Back Extention (Autodesk Fusion 360 design; units mm, degrees)
Autodesk Fusion 360 part; units mm, degrees
sketch "Sketch1" plane through (0, 0, 0) normal (0, 0, 1) x (1, 0, 0)
  line L0 (0, 0) -> (0, 121.8)
  line L1 (0, 0) -> (78.294095, 20.97884)
  line L2 (82, 25.808469) -> (82, 176.135475)
  line L3 (82, 176.135475) -> (44, 176.135475)
  line L4 (44, 176.135475) -> (0, 121.8)
  arc A0 (78.294095, 20.97884) -> (82, 25.808469) centre (77, 25.808469) ccw
  line L5 (3, 3.909676) -> (77.517638, 23.876617)
  arc A1 (77.517638, 23.876617) -> (79, 25.808469) centre (77, 25.808469) ccw
  line L6 (79, 25.808469) -> (79, 173.135475)
  line L7 (79, 173.135475) -> (45.430927, 173.135475)
  line L8 (45.430927, 173.135475) -> (3, 120.737644)
  line L9 (3, 3.909676) -> (3, 120.737644)
  line L10 (3, 91.254041) -> (79, 91.254041) construction
  line L11 (41, 167.663736) -> (41, 14.091745) construction
  circle A2 centre (41, 128.135475) radius 5
  circle A3 centre (41, 45) radius 5
  dimension "d3" = 121.8
  dimension "d4" = 75
  dimension "d5" = 141
  dimension "d6" = 82
  dimension "d7" = 75
  dimension "d8" = 38
  dimension "d9" = 5
  dimension "d64" = -3
  dimension "d86" = 10
  dimension "d87" = 45
  dimension "d88" = 10
  dimension "d89" = 45
  constraint coincident L0.start L1.start
  constraint vertical L0
  constraint parallel L0 L2
  constraint perpendicular L0 L3
  constraint tangent L2 A0
  constraint tangent L1 A0
  constraint perpendicular L6 L10
  constraint perpendicular L10 L11
  constraint coincident L11 A3.centre
  measures "d3" distance of L0.start L0.end
  measures "d4" angle of L0 L1
  measures "d5" angle of L0 L4
  measures "d6" distance of L0 L2
  measures "d7" angle of L0 L1
  measures "d9" radius of A0
  measures "d86" diameter of A2
  measures "d88" diameter of A3
  measures "d89" vertical distance of L0.start A3.centre
extrude "Extrude7" add sketch "Sketch1" along normal blind 3 contours L5 A1 L6 L7 L8 L9 | A2 | A3 picked at (67.925955, 108.535214) picked at (43.631771, 126.680026) picked at (42.542117, 43.337994) makes body 1
extrude "Extrude13" add sketch "Sketch1" along normal blind 45 contours L0 L1 L2 L3 L4 A0 | A2 | A3 picked at (81, 125.026473) picked at (43.631771, 126.680026) picked at (42.542117, 43.337994) bodies 1
sketch "Sketch2" plane through (0, 0, 0) normal (-1, 0, 0) x (0, -1, 0)
  line L0 (-121.8, 0) -> (0, 0)
  line L1 (0, 0) -> (0, 45)
  line L2 (0, 45) -> (-121.8, 45)
  line L3 (-121.8, 45) -> (-121.8, 0)
  line L4 (-45.9, 42) -> (-75.9, 42)
  line L5 (-75.9, 42) -> (-75.9, 6)
  line L6 (-75.9, 6) -> (-45.9, 6)
  line L7 (-45.9, 6) -> (-45.9, 42)
  line L8 (-45.9, 42) -> (-75.9, 6) construction
  line L9 (-75.9, 42) -> (-45.9, 6) construction
  line L10 (-60.9, 45) -> (-60.9, 0) construction
  line L11 (-30.9, 39) -> (-90.9, 39) construction
  line L12 (-90.9, 39) -> (-90.9, 9) construction
  line L13 (-90.9, 9) -> (-30.9, 9) construction
  line L14 (-30.9, 9) -> (-30.9, 39) construction
  line L15 (-30.9, 39) -> (-90.9, 9) construction
  line L16 (-90.9, 39) -> (-30.9, 9) construction
  circle A0 centre (-90.9, 9) radius 2.1
  circle A1 centre (-90.9, 39) radius 2.1
  circle A2 centre (-30.9, 9) radius 2.1
  circle A3 centre (-30.9, 39) radius 2.1
  line L17 (0, 29.417) -> (-121.8, 29.417) construction
  circle A4 centre (-10, 29.417) radius 5
  circle A5 centre (-111.8, 29.417) radius 5
  line L18 (-121.8, 0) -> (0, 0)
  line L19 (0, 0) -> (0, 45)
  line L20 (0, 45) -> (-121.8, 45)
  line L21 (-121.8, 45) -> (-121.8, 0)
  point P0 (-60.9, 24)
  point P1 (-60.9, 24)
  dimension "d16" = 30
  dimension "d17" = 36
  dimension "d19" = 60
  dimension "d20" = 30
  dimension "d21" = 4.2
  dimension "d22" = 4.2
  dimension "d23" = 4.2
  dimension "d24" = 4.2
  dimension "d26" = 50.9
  dimension "d27" = 10
  dimension "d54" = 30.9
  dimension "d55" = 90.9
  dimension "d67" = 29.417
  dimension "d68" = 6
  constraint horizontal L4
  constraint perpendicular L4 L5
  constraint parallel L4 L6
  constraint parallel L5 L7
  constraint coincident L8 P1
  constraint coincident L9 P1
  constraint midpoint L2 L10.start
  constraint midpoint L0 L10.end
  constraint coincident P1 L10
  constraint horizontal L11
  constraint perpendicular L11 L12
  constraint parallel L11 L13
  constraint parallel L12 L14
  constraint coincident L15 P1
  constraint coincident L16 P1
  constraint coincident P1 P0
  constraint coincident L12.end L13.start
  constraint coincident L11.end L12.start
  constraint coincident L13.end L14.start
  constraint coincident L11.start L14.end
  constraint coincident L1 L17.start
  constraint coincident L3 L17.end
  constraint perpendicular L3 L17
  constraint coincident L17 A4.centre
  constraint symmetric L10 A4 A5
  measures "d16" distance of L5.end L6.end
  measures "d17" distance of L4.end L5.end
  measures "d19" distance of L12.end L13.end
  measures "d20" distance of L11.end L12.end
  measures "d21" diameter of A0
  measures "d22" diameter of A1
  measures "d23" diameter of A2
  measures "d24" diameter of A3
  measures "d26" distance of L10 A4.centre
  measures "d27" diameter of A4
  measures "d54" horizontal distance of L0.end L13.end
  measures "d55" horizontal distance of L0.end L12.end
  measures "d67" distance of L0.end L17.start
  measures "d68" vertical distance of L0.end L6.end
extrude "Extrude16" cut sketch "Sketch2" against normal blind 10 contours L4 L5 L6 L7 | A0 | A1 | A2 | A3 | A4 | A5 picked at (-65.9, 18) picked at (-90.207818, 8.89567) picked at (-91.354622, 39.606218) picked at (-32.17464, 9.251722) picked at (-31.534769, 38.918203) picked at (-10.833333, 30.579729) picked at (-113.210608, 28.925741) bodies 1
sketch "Sketch3" plane through (0, 176.135475, 0) normal (0, 1, 0) x (-1, 0, 0)
  line L0 (-82, 0) -> (-44, 0)
  line L1 (-44, 0) -> (-44, 45)
  line L2 (-44, 45) -> (-82, 45)
  line L3 (-82, 45) -> (-82, 0)
  line L4 (-44, 45) -> (-82, 0) construction
  line L5 (-50.5, 7.5) -> (-75.5, 7.5) construction
  line L6 (-75.5, 7.5) -> (-75.5, 37.5) construction
  line L7 (-75.5, 37.5) -> (-50.5, 37.5) construction
  line L8 (-50.5, 37.5) -> (-50.5, 7.5) construction
  line L9 (-50.5, 7.5) -> (-75.5, 37.5) construction
  line L10 (-75.5, 7.5) -> (-50.5, 37.5) construction
  circle A0 centre (-75.5, 37.5) radius 1.6
  circle A1 centre (-50.5, 37.5) radius 1.6
  circle A2 centre (-75.5, 7.5) radius 1.6
  circle A3 centre (-50.5, 7.5) radius 1.6
  circle A4 centre (-63, 22.5) radius 12.5
  line L11 (-82, 0) -> (-44, 0)
  line L12 (-44, 0) -> (-44, 45)
  line L13 (-44, 45) -> (-82, 45)
  line L14 (-82, 45) -> (-82, 0)
  point P0 (-63, 22.5)
  dimension "d30" = 3.2
  dimension "d31" = 3.2
  dimension "d32" = 3.2
  dimension "d33" = 3.2
  dimension "d34" = 25
  dimension "d35" = 30
  dimension "d36" = 25
  constraint coincident L1.end L2.start
  constraint coincident L0.start L3.end
  constraint horizontal L5
  constraint perpendicular L5 L6
  constraint parallel L5 L7
  constraint parallel L6 L8
  constraint coincident L9 P0
  constraint coincident L10 P0
  constraint midpoint L4 P0
  constraint coincident L6.end L7.start
  constraint coincident L7.end L8.start
  constraint coincident L5.end L6.start
  constraint coincident L5.start L8.end
  constraint coincident P0 A4.centre
  measures "d30" diameter of A0
  measures "d31" diameter of A1
  measures "d32" diameter of A2
  measures "d33" diameter of A3
  measures "d34" distance of L6.end L7.end
  measures "d35" distance of L5.end L6.end
  measures "d36" diameter of A4
extrude "Extrude17" cut sketch "Sketch3" against normal blind 10 contours A0 | A1 | A2 | A3 | A4 picked at (-75.766667, 36.57531) picked at (-50.233333, 38.276286) picked at (-75.167472, 8.379786) picked at (-50.167472, 8.231382) picked at (-57.779901, 21.179037) bodies 1
sketch "Sketch5" plane through (0, 0, 45) normal (0, 0, 1) x (-1, 0, 0)
  circle A0 centre (-41, -45) radius 5
  circle A1 centre (-41, -128.135475) radius 5
  circle A2 centre (-41, -128.135475) radius 0.75
  circle A3 centre (-41, -45) radius 0.75
  circle A4 centre (-41, -45) radius 5
  dimension "d90" = 1.5
  dimension "d91" = 1.5
  constraint concentric A1 A2
  constraint concentric A0 A3
  measures "d90" diameter of A2
  measures "d91" diameter of A3
fillet "Fillet2" radius 2.5 6 edges at (3, 62.32366, 3) (24.215463, 146.93656, 3) (62.215463, 173.135475, 3) (40.258819, 13.893147, 3) (78.586707, 24.590946, 3) (79, 99.471972, 3) on bodies 1
fillet "Fillet2" radius 2.5 2 edges at (36.338363, 129.943552, 3) (36.338363, 46.808077, 3) on bodies 1
extrude "Extrude14" cut 2 faces at (42.542117, 43.337994, 45) (43.631771, 126.680026, 45) along direction (0, 0, -1) blind 3 on bodies 1 bodies 1
extrude "Extrude15" cut sketch "Sketch5" against normal blind 20 contours A2 | A3 picked at (-41.367375, -128.379207) picked at (-40.981317, -45.101923) bodies 1
sketch "Sketch4" plane through (0, 0, 45) normal (0, 0, 1) x (1, 0, 0)
  arc A0 (77.517638, 23.876617) -> (79, 25.808469) centre (77, 25.808469) ccw
  line L0 (77.517638, 23.876617) -> (3, 3.909676)
  line L1 (3, 3.909676) -> (3, 120.737644)
  line L2 (3, 120.737644) -> (45.430927, 173.135475)
  line L3 (45.430927, 173.135475) -> (79, 173.135475)
  line L4 (79, 173.135475) -> (79, 25.808469)
  line L5 (0, 0) -> (78.294095, 20.97884)
  arc A1 (78.294095, 20.97884) -> (82, 25.808469) centre (77, 25.808469) ccw
  line L6 (82, 25.808469) -> (82, 176.135475)
  line L7 (82, 176.135475) -> (44, 176.135475)
  line L8 (44, 176.135475) -> (0, 121.8)
  line L9 (0, 121.8) -> (0, 0)
  line L10 (3, 106.572901) -> (3, 10.425803)
  line L11 (11.914162, 131.745717) -> (42.429222, 169.428679)
  line L12 (50.200682, 173.135475) -> (74, 173.135475)
  line L13 (79, 168.135475) -> (79, 31.947085)
  line L14 (9.294095, 5.596174) -> (71.58819, 22.287826)
  arc A2 (11.914162, 131.745717) -> (3, 106.572901) centre (43, 106.572901) ccw
  arc A3 (50.200682, 173.135475) -> (42.429222, 169.428679) centre (50.200682, 163.135475) ccw
  arc A4 (79, 168.135475) -> (74, 173.135475) centre (74, 168.135475) ccw
  arc A5 (3, 10.425803) -> (9.294095, 5.596174) centre (8, 10.425803) ccw
  arc A6 (71.58819, 22.287826) -> (79, 31.947085) centre (69, 31.947085) ccw
  line L15 (13, 27.309676) -> (3, 27.309676)
  line L16 (3, 27.309676) -> (3, 42.309676)
  line L17 (3, 42.309676) -> (13, 42.309676)
  line L18 (13, 42.309676) -> (13, 27.309676)
  line L19 (13, 27.309676) -> (3, 42.309676) construction
  line L20 (3, 27.309676) -> (13, 42.309676) construction
  line L21 (13, 87.309676) -> (3, 87.309676)
  line L22 (3, 87.309676) -> (3, 102.309676)
  line L23 (3, 102.309676) -> (13, 102.309676)
  line L24 (13, 102.309676) -> (13, 87.309676)
  line L25 (13, 87.309676) -> (3, 102.309676) construction
  line L26 (3, 87.309676) -> (13, 102.309676) construction
  arc A7 (77.517638, 23.876617) -> (79, 25.808469) centre (77, 25.808469) ccw
  line L27 (77.517638, 23.876617) -> (3, 3.909676)
  line L28 (3, 3.909676) -> (3, 120.737644)
  line L29 (3, 120.737644) -> (45.430927, 173.135475)
  line L30 (45.430927, 173.135475) -> (79, 173.135475)
  line L31 (79, 173.135475) -> (79, 25.808469)
  line L32 (0, 0) -> (78.294095, 20.97884)
  arc A8 (78.294095, 20.97884) -> (82, 25.808469) centre (77, 25.808469) ccw
  line L33 (82, 25.808469) -> (82, 176.135475)
  line L34 (82, 176.135475) -> (44, 176.135475)
  line L35 (44, 176.135475) -> (0, 121.8)
  line L36 (0, 121.8) -> (0, 0)
  circle A9 centre (41, 128.135475) radius 0.75
  circle A10 centre (41, 45) radius 0.75
  circle A11 centre (41, 128.135475) radius 1.75
  circle A12 centre (41, 45) radius 1.75
  point P0 (8, 34.809676)
  point P1 (8, 94.809676)
  dimension "d69" = 40
  dimension "d70" = 10
  dimension "d71" = 5
  dimension "d72" = 5
  dimension "d73" = 10
  dimension "d74" = 10
  dimension "d75" = 15
  dimension "d76" = 10
  dimension "d77" = 15
  dimension "d78" = 30.9
  dimension "d79" = 90.9
  dimension "d108" = 3.5
  dimension "d109" = 3.5
  constraint tangent L11 A2
  constraint tangent L10 A2
  constraint tangent L11 A3
  constraint tangent L12 A3
  constraint tangent L12 A4
  constraint tangent L13 A4
  constraint tangent L10 A5
  constraint tangent L14 A5
  constraint tangent L14 A6
  constraint tangent L13 A6
  constraint horizontal L15
  constraint perpendicular L15 L16
  constraint parallel L15 L17
  constraint parallel L16 L18
  constraint horizontal L21
  constraint perpendicular L21 L22
  constraint parallel L21 L23
  constraint parallel L22 L24
  constraint concentric A9 A11
  constraint concentric A10 A12
  measures "d69" radius of A2
  measures "d70" radius of A3
  measures "d71" radius of A4
  measures "d72" radius of A5
  measures "d73" radius of A6
  measures "d108" diameter of A11
  measures "d109" diameter of A12
extrude "Extrude8" add sketch "Sketch4" against normal blind 3 separate body contours L0 L1 L2 L3 L4 L10 L11 L12 L13 L14 A2 A3 A4 A5 A6 L15 L17 L18 L21 L23 L24 L27 L28 L29 L30 L31 picked at (66.866235, 109.168748) makes body 2
extrude "Extrude10" add sketch "Sketch4" along normal blind 1 contours A0 L0 L4 A6 A7 L27 L31 | L0 L1 L2 L3 L4 L10 L11 L12 L13 L14 A2 A3 A4 A5 A6 L15 L17 L18 L21 L23 L24 L27 L28 L29 L30 L31 | L0 L1 A5 L27 L28 | L3 L4 A4 L30 L31 | L1 L10 L15 L16 L17 L18 L28 | L2 L3 A3 L29 L30 | L1 L10 L21 L22 L23 L24 L28 | L1 L2 A2 L28 L29 | L5 A1 L6 L7 L8 L9 L32 A8 L33 L34 L35 L36 picked at (77.498701, 25.486857) picked at (66.866235, 109.168748) picked at (4.309167, 5.615816) picked at (78.017684, 172.153159) picked at (6.333333, 37.309676) picked at (46.201154, 172.665108) picked at (6.333333, 97.309676) picked at (4.587771, 120.175385) picked at (1, 49.703225) bodies 2
mirror "Mirror3" about plane through (0, 0, 0) normal (1, 0, 0) of bodies 1 makes body 3
move_body "Move5" bodies 3 to x (1, 0, 0) y (0, 1, 0) z (0, 0, 1) at (-50, 0, 0)
mirror "Mirror4" about plane through (0, 0, 0) normal (1, 0, 0) of bodies 2 makes body 4
move_body "Move6" bodies 4 to x (1, 0, 0) y (0, 1, 0) z (0, 0, 1) at (-50, 0, 0)
copy_body "Body->Comp1" bodies 1 removing the originals makes body 5 in component "Back Ext - Right"
copy_body "Body->Comp2" bodies 2 removing the originals makes body 6 in component "Back Ext Cover - Right"
copy_body "Body->Comp3" bodies 3 removing the originals makes body 7 in component "Back Ext - Left"
copy_body "Body->Comp4" bodies 4 removing the originals makes body 8 in component "Back Ext Cover - Left"
component "Back Ext - Right" placed x (1, 0, 0) y (0, 1, 0) z (0, 0, 1) at (0, 0, 0)
component "Back Ext Cover - Right" placed x (1, 0, 0) y (0, 1, 0) z (0, 0, 1) at (0, 0, 0)
component "Back Ext - Left" placed x (1, 0, 0) y (0, 1, 0) z (0, 0, 1) at (0, 0, 0)
component "Back Ext Cover - Left" placed x (1, 0, 0) y (0, 1, 0) z (0, 0, 1) at (0, 0, 0)
equation "d26 = ( 101.8 / 2 ) * 1 mm"
named bodies: "Back2 - Right", "Back - Right", "Back - Left", "Back2 - Left"
